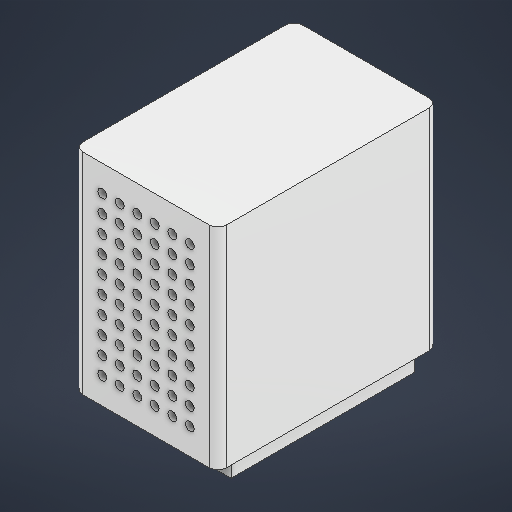
# Autodesk Inventor part: encloser-dht22_command
Saved by Autodesk Inventor 2025.2 (Build 292293000, 293)
## iProperties
Created: 2026-01-02
Part Number: encloser-dht22_command
Material: PC/ABS Plastic
Document SubType Name: Modeling
Designer: sam
Density: 1.1 g/cm^3
Appearance: Smooth - White
Author: sam
Autodesk Inventor part; units mm, degrees
ref_plane "YZ Plane" through (0, 0, 0) normal (1, 0, 0) x (0, 1, 0)
ref_plane "XZ Plane" through (0, 0, 0) normal (0, 1, 0) x (-1, 0, 0)
ref_plane "XY Plane" through (0, 0, 0) normal (0, 0, 1) x (1, 0, 0)
sketch "Sketch1" plane through (0, 0, 0) normal (0, 1, 0) x (-1, 0, 0)
  line L0 (8.2, 12.55) -> (-8.2, 12.55)
  line L1 (-8.2, 12.55) -> (-8.2, -12.55)
  line L2 (-8.2, -12.55) -> (8.2, -12.55)
  line L3 (8.2, -12.55) -> (8.2, 12.55)
  line L4 (8.2, 12.55) -> (-8.2, -12.55) construction
  line L5 (-8.2, 12.55) -> (8.2, -12.55) construction
  point P0 (0, 0)
  dimension "d0" = 16.4
  dimension "d1" = 25.1
  constraints: 12 end point, 2 midpoint, 2 parallel, 1 horizontal, 1 perpendicular
  measures "d0" distance of L2.end L1.end
  measures "d1" distance of L1.end L0.end
extrude "Extrusion1" add sketch "Sketch1" against normal blind 2
sketch "Sketch2" plane through (0, -2, 0) normal (0, -1, 0) x (1, 0, 0)
  line L0 (8.2, -12.55) -> (8.2, 12.55) projected
  line L1 (8.2, 12.55) -> (-8.2, 12.55) projected
  line L2 (-8.2, 12.55) -> (-8.2, -12.55) projected
  line L3 (-8.2, -12.55) -> (8.2, -12.55) projected
  line L4 (8.2, 12.55) -> (5.2, 12.55)
  line L5 (5.2, 12.55) -> (5.2, -12.55)
  line L6 (5.2, -12.55) -> (8.2, -12.55)
  line L7 (8.2, -12.55) -> (8.2, 12.55)
  line L8 (-8.2, -12.55) -> (-5.2, -12.55)
  line L9 (-5.2, -12.55) -> (-5.2, 12.55)
  line L10 (-5.2, 12.55) -> (-8.2, 12.55)
  line L11 (-8.2, 12.55) -> (-8.2, -12.55)
  line L12 (-5.2, 12.55) -> (5.2, 12.55)
  line L13 (5.2, 12.55) -> (5.2, 11.55)
  line L14 (5.2, 11.55) -> (-5.2, 11.55)
  line L15 (-5.2, 11.55) -> (-5.2, 12.55)
  line L16 (-5.2, -12.55) -> (5.2, -12.55)
  line L17 (5.2, -12.55) -> (5.2, -11.55)
  line L18 (5.2, -11.55) -> (-5.2, -11.55)
  line L19 (-5.2, -11.55) -> (-5.2, -12.55)
  point P0 (0, 0)
  point P1 (-5.2, 11.55)
  dimension "d4" = 3
  dimension "d5" = 3
  dimension "d6" = 1
  dimension "d7" = 1
  constraints: 32 end point, 8 parallel, 4 horizontal, 4 perpendicular, 4 point on line
  measures "d4" distance of L6.end L5.end
  measures "d5" distance of L10.end L9.end
  measures "d6" distance of L12.end L13.end
  measures "d7" distance of L17.end L16.end
extrude "Extrusion2" add sketch "Sketch2" along normal blind 22 contours L3 L5 L1 L0 | L3 L9 L18 L5 | L5 L14 L9 L1 | L3 L2 L1 L9
sketch "Sketch3" plane through (0, -24, 0) normal (0, -1, 0) x (1, 0, 0)
  line L0 (-7.6, 10.45) -> (-5.8, 10.45)
  line L1 (-5.8, 10.45) -> (-5.8, -10.45)
  line L2 (-5.8, -10.45) -> (-7.6, -10.45)
  line L3 (-7.6, -10.45) -> (-7.6, 10.45)
  line L4 (5.8, 10.45) -> (7.6, 10.45)
  line L5 (7.6, 10.45) -> (7.6, -10.45)
  line L6 (7.6, -10.45) -> (5.8, -10.45)
  line L7 (5.8, -10.45) -> (5.8, 10.45)
  line L8 (5.2, 11.55) -> (5.2, -11.55) projected
  line L9 (-5.2, -11.55) -> (-5.2, 11.55) projected
  line L10 (5.2, -11.55) -> (-5.2, -11.55) projected
  line L11 (-5.2, 11.55) -> (5.2, 11.55) projected
  point P0 (0, 0)
  dimension "d10" = 1.8
  dimension "d11" = 1.8
  dimension "d12" = 0.6
  dimension "d13" = 0.6
  dimension "d14" = 1.1
  dimension "d15" = 1.1
  dimension "d16" = 1.1
  dimension "d17" = 1.1
  constraints: 16 end point, 4 parallel, 2 horizontal, 2 perpendicular
  measures "d10" distance of L1.end L2.end
  measures "d11" distance of L5.end L6.end
  measures "d12" distance between parallel lines of L8 L7
  measures "d13" distance between parallel lines of L9 L1
  measures "d14" distance between parallel lines of L10 L2
  measures "d15" distance between parallel lines of L6 L10
  measures "d16" distance between parallel lines of L11 L4
  measures "d17" distance between parallel lines of L11 L0
extrude "Extrusion3" add sketch "Sketch3" along normal blind 1.9 contours L0 L1 L2 L3 | L4 L5 L6 L7
sketch "Sketch4" plane through (-8.2, 0, -12.55) normal (-1, 0, 0) x (0, 0, 1)
  line L0 (0, 0) -> (25.1, 0) projected
  line L1 (0, 0) -> (0, -24) projected
  line L2 (25.1, -24) -> (0, -24) projected
  line L3 (25.1, 0) -> (25.1, -24) projected
  circle A0 centre (2.55, -3) radius 0.5
  circle A1 centre (4.55, -3) radius 0.5
  circle A2 centre (6.55, -3) radius 0.5
  circle A3 centre (8.55, -3) radius 0.5
  circle A4 centre (10.55, -3) radius 0.5
  circle A5 centre (12.55, -3) radius 0.5
  circle A6 centre (14.55, -3) radius 0.5
  circle A7 centre (16.55, -3) radius 0.5
  circle A8 centre (18.55, -3) radius 0.5
  circle A9 centre (20.55, -3) radius 0.5
  circle A10 centre (22.55, -3) radius 0.5
  circle A11 centre (2.55, -5) radius 0.5
  circle A12 centre (4.55, -5) radius 0.5
  circle A13 centre (6.55, -5) radius 0.5
  circle A14 centre (8.55, -5) radius 0.5
  circle A15 centre (10.55, -5) radius 0.5
  circle A16 centre (12.55, -5) radius 0.5
  circle A17 centre (14.55, -5) radius 0.5
  circle A18 centre (16.55, -5) radius 0.5
  circle A19 centre (18.55, -5) radius 0.5
  circle A20 centre (20.55, -5) radius 0.5
  circle A21 centre (22.55, -5) radius 0.5
  circle A22 centre (2.55, -7) radius 0.5
  circle A23 centre (4.55, -7) radius 0.5
  circle A24 centre (6.55, -7) radius 0.5
  circle A25 centre (8.55, -7) radius 0.5
  circle A26 centre (10.55, -7) radius 0.5
  circle A27 centre (12.55, -7) radius 0.5
  circle A28 centre (14.55, -7) radius 0.5
  circle A29 centre (16.55, -7) radius 0.5
  circle A30 centre (18.55, -7) radius 0.5
  circle A31 centre (20.55, -7) radius 0.5
  circle A32 centre (22.55, -7) radius 0.5
  circle A33 centre (2.55, -9) radius 0.5
  circle A34 centre (4.55, -9) radius 0.5
  circle A35 centre (6.55, -9) radius 0.5
  circle A36 centre (8.55, -9) radius 0.5
  circle A37 centre (10.55, -9) radius 0.5
  circle A38 centre (12.55, -9) radius 0.5
  circle A39 centre (14.55, -9) radius 0.5
  circle A40 centre (16.55, -9) radius 0.5
  circle A41 centre (18.55, -9) radius 0.5
  circle A42 centre (20.55, -9) radius 0.5
  circle A43 centre (22.55, -9) radius 0.5
  circle A44 centre (2.55, -11) radius 0.5
  circle A45 centre (4.55, -11) radius 0.5
  circle A46 centre (6.55, -11) radius 0.5
  circle A47 centre (8.55, -11) radius 0.5
  circle A48 centre (10.55, -11) radius 0.5
  circle A49 centre (12.55, -11) radius 0.5
  circle A50 centre (14.55, -11) radius 0.5
  circle A51 centre (16.55, -11) radius 0.5
  circle A52 centre (18.55, -11) radius 0.5
  circle A53 centre (20.55, -11) radius 0.5
  circle A54 centre (22.55, -11) radius 0.5
  circle A55 centre (2.55, -13) radius 0.5
  circle A56 centre (4.55, -13) radius 0.5
  circle A57 centre (6.55, -13) radius 0.5
  circle A58 centre (8.55, -13) radius 0.5
  circle A59 centre (10.55, -13) radius 0.5
  circle A60 centre (12.55, -13) radius 0.5
  circle A61 centre (14.55, -13) radius 0.5
  circle A62 centre (16.55, -13) radius 0.5
  circle A63 centre (18.55, -13) radius 0.5
  circle A64 centre (20.55, -13) radius 0.5
  circle A65 centre (22.55, -13) radius 0.5
  circle A66 centre (2.55, -15) radius 0.5
  circle A67 centre (4.55, -15) radius 0.5
  circle A68 centre (6.55, -15) radius 0.5
  circle A69 centre (8.55, -15) radius 0.5
  circle A70 centre (10.55, -15) radius 0.5
  circle A71 centre (12.55, -15) radius 0.5
  circle A72 centre (14.55, -15) radius 0.5
  circle A73 centre (16.55, -15) radius 0.5
  circle A74 centre (18.55, -15) radius 0.5
  circle A75 centre (20.55, -15) radius 0.5
  circle A76 centre (22.55, -15) radius 0.5
  circle A77 centre (2.55, -17) radius 0.5
  circle A78 centre (4.55, -17) radius 0.5
  circle A79 centre (6.55, -17) radius 0.5
  circle A80 centre (8.55, -17) radius 0.5
  circle A81 centre (10.55, -17) radius 0.5
  circle A82 centre (12.55, -17) radius 0.5
  circle A83 centre (14.55, -17) radius 0.5
  circle A84 centre (16.55, -17) radius 0.5
  circle A85 centre (18.55, -17) radius 0.5
  circle A86 centre (20.55, -17) radius 0.5
  circle A87 centre (22.55, -17) radius 0.5
  circle A88 centre (2.55, -19) radius 0.5
  circle A89 centre (4.55, -19) radius 0.5
  circle A90 centre (6.55, -19) radius 0.5
  circle A91 centre (8.55, -19) radius 0.5
  circle A92 centre (10.55, -19) radius 0.5
  circle A93 centre (12.55, -19) radius 0.5
  circle A94 centre (14.55, -19) radius 0.5
  circle A95 centre (16.55, -19) radius 0.5
  circle A96 centre (18.55, -19) radius 0.5
  circle A97 centre (20.55, -19) radius 0.5
  circle A98 centre (22.55, -19) radius 0.5
  circle A99 centre (2.55, -21) radius 0.5
  circle A100 centre (4.55, -21) radius 0.5
  circle A101 centre (6.55, -21) radius 0.5
  circle A102 centre (8.55, -21) radius 0.5
  circle A103 centre (10.55, -21) radius 0.5
  circle A104 centre (12.55, -21) radius 0.5
  circle A105 centre (14.55, -21) radius 0.5
  circle A106 centre (16.55, -21) radius 0.5
  circle A107 centre (18.55, -21) radius 0.5
  circle A108 centre (20.55, -21) radius 0.5
  circle A109 centre (22.55, -21) radius 0.5
  point P0 (12.55, 0)
  dimension "d20" = 1
  dimension "d21" = 2.55
  dimension "d22" = 3
  dimension "d25" = 2
  dimension "d28" = 2
  constraints: 110 centre point, 1 horizontal, 1 vertical, 218 other
  measures "d20" diameter of A0
  measures "d21" distance from line of L1 A0.centre
  measures "d22" distance from line of L0 A0.centre
  measures "d25" distance of A0.centre A1.centre
  measures "d28" distance of A0.centre A11.centre
extrude "Extrusion4" cut sketch "Sketch4" against normal blind 3 contours A0 | A1 | A2 | A3 | A4 | A5 | A6 | A7 | A8 | A9 | A10 | A11 | A12 | A13 | A14 | A15 | A16 | A17 | A18 | A19 | A20 | A21 | A22 | A23 | A24 | A25 | A26 | A27 | A28 | A29 | A30 | A31 | A32 | A33 | A34 | A35 | A36 | A37 | A38 | A39 | A40 | A41 | A42 | A43 | A44 | A45 | A46 | A47 | A48 | A49 | A50 | A51 | A52 | A53 | A54 | A55 | A56 | A57 | A58 | A59 | A60 | A61 | A62 | A63 | A64 | A65 | A66 | A67 | A68 | A69 | A70 | A71 | A72 | A73 | A74 | A75 | A76 | A77 | A78 | A79 | A80 | A81 | A82 | A83 | A84 | A85 | A86 | A87 | A88 | A89 | A90 | A91 | A92 | A93 | A94 | A95 | A96 | A97 | A98 | A99 | A100 | A101 | A102 | A103 | A104 | A105 | A106 | A107 | A108 | A109
fillet "Fillet2" radius 1 4 edges at (8.2, -12, 12.55) (-8.2, -12, 12.55) (8.2, -12, -12.55) (-8.2, -12, -12.55)
sketch "Sketch5" plane through (-7.2, 0, 12.55) normal (0, 0, 1) x (1, 0, 0)
  circle A0 centre (2.2, -3) radius 0.5
  line L0 (0, -24) -> (0, 0) projected
  line L1 (14.4, -24) -> (0, -24) projected
  line L2 (14.4, 0) -> (14.4, -24) projected
  line L3 (0, 0) -> (14.4, 0) projected
  circle A1 centre (4.2, -3) radius 0.5
  circle A2 centre (6.2, -3) radius 0.5
  circle A3 centre (8.2, -3) radius 0.5
  circle A4 centre (10.2, -3) radius 0.5
  circle A5 centre (2.2, -5) radius 0.5
  circle A6 centre (4.2, -5) radius 0.5
  circle A7 centre (6.2, -5) radius 0.5
  circle A8 centre (8.2, -5) radius 0.5
  circle A9 centre (10.2, -5) radius 0.5
  circle A10 centre (2.2, -7) radius 0.5
  circle A11 centre (4.2, -7) radius 0.5
  circle A12 centre (6.2, -7) radius 0.5
  circle A13 centre (8.2, -7) radius 0.5
  circle A14 centre (10.2, -7) radius 0.5
  circle A15 centre (2.2, -9) radius 0.5
  circle A16 centre (4.2, -9) radius 0.5
  circle A17 centre (6.2, -9) radius 0.5
  circle A18 centre (8.2, -9) radius 0.5
  circle A19 centre (10.2, -9) radius 0.5
  circle A20 centre (2.2, -11) radius 0.5
  circle A21 centre (4.2, -11) radius 0.5
  circle A22 centre (6.2, -11) radius 0.5
  circle A23 centre (8.2, -11) radius 0.5
  circle A24 centre (10.2, -11) radius 0.5
  circle A25 centre (2.2, -13) radius 0.5
  circle A26 centre (4.2, -13) radius 0.5
  circle A27 centre (6.2, -13) radius 0.5
  circle A28 centre (8.2, -13) radius 0.5
  circle A29 centre (10.2, -13) radius 0.5
  circle A30 centre (2.2, -15) radius 0.5
  circle A31 centre (4.2, -15) radius 0.5
  circle A32 centre (6.2, -15) radius 0.5
  circle A33 centre (8.2, -15) radius 0.5
  circle A34 centre (10.2, -15) radius 0.5
  circle A35 centre (2.2, -17) radius 0.5
  circle A36 centre (4.2, -17) radius 0.5
  circle A37 centre (6.2, -17) radius 0.5
  circle A38 centre (8.2, -17) radius 0.5
  circle A39 centre (10.2, -17) radius 0.5
  circle A40 centre (2.2, -19) radius 0.5
  circle A41 centre (4.2, -19) radius 0.5
  circle A42 centre (6.2, -19) radius 0.5
  circle A43 centre (8.2, -19) radius 0.5
  circle A44 centre (10.2, -19) radius 0.5
  circle A45 centre (2.2, -21) radius 0.5
  circle A46 centre (4.2, -21) radius 0.5
  circle A47 centre (6.2, -21) radius 0.5
  circle A48 centre (8.2, -21) radius 0.5
  circle A49 centre (10.2, -21) radius 0.5
  circle A50 centre (12.2, -3) radius 0.5
  circle A51 centre (12.2, -5) radius 0.5
  circle A52 centre (12.2, -7) radius 0.5
  circle A53 centre (12.2, -9) radius 0.5
  circle A54 centre (12.2, -11) radius 0.5
  circle A55 centre (12.2, -13) radius 0.5
  circle A56 centre (12.2, -15) radius 0.5
  circle A57 centre (12.2, -17) radius 0.5
  circle A58 centre (12.2, -19) radius 0.5
  circle A59 centre (12.2, -21) radius 0.5
  point P0 (7.2, 0)
  dimension "d35" = 1
  dimension "d38" = 2
  dimension "d41" = 2
  dimension "d44" = 3
  dimension "d45" = 2.2
  constraints: 60 centre point, 1 horizontal, 1 vertical, 118 other
  measures "d35" diameter of A0
  measures "d38" distance of A0.centre A1.centre
  measures "d41" distance of A0.centre A5.centre
  measures "d44" distance from line of L3 A0.centre
  measures "d45" distance from line of L0 A0.centre
extrude "Extrusion5" cut sketch "Sketch5" against normal through all contours A0 | A1 | A2 | A3 | A4 | A5 | A6 | A7 | A8 | A9 | A10 | A11 | A12 | A13 | A14 | A15 | A16 | A17 | A18 | A19 | A20 | A21 | A22 | A23 | A24 | A25 | A26 | A27 | A28 | A29 | A30 | A31 | A32 | A33 | A34 | A35 | A36 | A37 | A38 | A39 | A40 | A41 | A42 | A43 | A44 | A45 | A46 | A47 | A48 | A49 | A50 | A51 | A52 | A53 | A54 | A55 | A56 | A57 | A58 | A59
body "Solid1"
